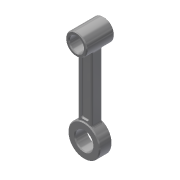
# Autodesk Inventor part: Connector Arm1
Saved by Autodesk Inventor 2022 Beta2 (Build 260130000, 130) ContinuousBuild 0
## iProperties
Shininess: 64.0
Angle Display Precision: 2
Document Length Units: 11272
Document Angle Units: 11279
Document Time Units: 11290
Document Mass Units: 11286
Document Length Units Precision: 3
Document Angle Units Precision: 2
Created: 2002-04-22
Part Number: Connector Arm1
Material: Stainless Steel, Austenitic
Document SubType Name: Modeling
Designer: Nino
Density: 8.03 g/cm^3
Appearance: Steel
Density: 0.0
Volumn: 0.0
Area: 0.0
PropertySet Name: Model Information
Control State: 0
Master: False
Checked Out: False
Author: Nino
Autodesk Inventor part; units mm, degrees
ref_plane "YZ Plane" through (0, 0, 0) normal (1, 0, 0) x (0, 1, 0)
ref_plane "XZ Plane" through (0, 0, 0) normal (0, 1, 0) x (-1, 0, 0)
sketch "Sketch1" plane through (0, 0, 0) normal (0, 0, 1) x (1, 0, 0)
  line L0 (416.0385, 369.5119) -> (416.0385, 213.9034)
  circle A0 centre (416.0385, 369.5119) radius 12.7
  circle A1 centre (416.0385, 213.9034) radius 15.875
  circle A2 centre (416.0385, 369.5119) radius 19.05
  circle A3 centre (416.0385, 213.9034) radius 28.575
  line L1 (428.7385, 355.3128) -> (428.7385, 239.5011)
  line L2 (403.3385, 355.3128) -> (403.3385, 239.5011)
  dimension "d0" = 25.4
  dimension "d1" = 31.75
  dimension "d2" = 6.35
  dimension "d3" = 12.7
  dimension "d4" = 12.7
  dimension "d5" = 12.7
  dimension "d6" = 155.6085
  constraints: 6 end point, 4 centre point, 4 point on circle, 2 coincident, 1 vertical
  measures "d0" diameter of A0
  measures "d1" diameter of A1
  measures "d2" radial gap between concentric circles of A2 A0
  measures "d3" radial gap between concentric circles of A3 A1
  measures "d4" distance between parallel lines of L2 L0
  measures "d5" distance between parallel lines of L1 L0
  measures "d6" distance of L0.start L0.end
extrude "Extrusion1" add sketch "Sketch1" along normal mid plane 19.05
ref_plane "Work Plane1" through (0, 0, 0) normal (0, 0, 1) x (1, 0, 0)
sketch "Sketch2" plane through (0, 0, 0) normal (0, 0, 1) x (1, 0, 0)
  circle A0 centre (416.0385, 369.5119) radius 12.7
  circle A1 centre (416.0385, 213.9034) radius 15.875
  circle A2 centre (416.0385, 369.5119) radius 19.05
  circle A3 centre (416.0385, 213.9034) radius 28.575
  point P0 (428.7385, 355.3128)
  point P1 (428.7385, 239.5011)
  point P2 (403.3385, 355.3128)
  point P3 (403.3385, 239.5011)
  dimension "d10" = 25.4
  dimension "d11" = 31.75
  dimension "d12" = 6.35
  dimension "d13" = 12.7
  constraints: 4 centre point, 4 point on circle
  measures "d10" diameter of A0
  measures "d11" diameter of A1
  measures "d12" radial gap between concentric circles of A2 A0
  measures "d13" radial gap between concentric circles of A3 A1
extrude "Extrusion2" add sketch "Sketch2" along normal mid plane 49.53 contours A2
extrude "Extrusion3" add sketch "Sketch2" along normal mid plane 22.352 contours A3
chamfer "Chamfer1" distance 1.524 angle 45 8 edges at (403.3385, 369.5119, 24.765) (396.9885, 369.5119, 24.765) (396.9885, 369.5119, -24.765) (403.3385, 369.5119, -24.765) (387.4635, 213.9034, 11.176) (400.1635, 213.9034, 11.176) (387.4635, 213.9034, -11.176) (400.1635, 213.9034, -11.176)
fillet "Fillet1" radius 6.35 6 edges at (428.7385, 355.3128, 0) (403.3385, 355.3128, 0) (403.3385, 239.5011, 4.7625) (403.3385, 239.5011, -4.7625) (428.7385, 239.5011, 4.7625) (428.7385, 239.5011, -4.7625)
fillet "Fillet2" radius 3.175 12 edges at (403.3385, 297.9434, 9.525) (402.9284, 354.9564, 9.525) (402.5705, 240.1482, 9.525) (403.3385, 297.9434, -9.525) (402.5705, 240.1482, -9.525) (402.9284, 354.9564, -9.525) (428.7385, 297.9434, 9.525) (429.5066, 240.1482, 9.525) (429.1487, 354.9564, 9.525) (428.7385, 297.9434, -9.525) (429.1487, 354.9564, -9.525) (429.5066, 240.1482, -9.525)
sketch "Sketch3" plane through (0, 0, 9.525) normal (0, 0, 1) x (1, 0, 0)
  arc A0 (406.5086, 353.0169) -> (425.5684, 353.0169) centre (416.0385, 369.5119) ccw projected
  line L0 (406.5135, 243.1755) -> (406.5135, 352.7114) projected
  line L1 (425.5635, 352.7114) -> (425.5635, 243.1755) projected
  line L2 (409.0535, 347.1599) -> (423.0235, 347.1599)
  line L3 (423.0235, 347.1599) -> (423.0235, 245.6534)
  line L4 (423.0235, 245.6534) -> (409.0535, 245.6534)
  line L5 (409.0535, 245.6534) -> (409.0535, 347.1599)
  circle A1 centre (416.0385, 213.9034) radius 17.399 projected
  dimension "d22" = 22.352
  dimension "d23" = 31.75
  dimension "d24" = 2.54
  dimension "d25" = 2.54
  constraints: 8 end point, 2 parallel, 1 horizontal, 1 perpendicular
  measures "d22" distance from line of A0.centre L2
  measures "d23" distance from line of A1.centre L4
  measures "d24" distance between parallel lines of L0 L5
  measures "d25" distance between parallel lines of L1 L3
extrude "Extrusion4" cut sketch "Sketch3" against normal blind 3.175 contours L2 L3 L4 L5
fillet "Fillet3" radius 3.175 4 edges at (409.0535, 245.6534, 7.9375) (423.0235, 245.6534, 7.9375) (409.0535, 347.1599, 7.9375) (423.0235, 347.1599, 7.9375)
fillet "Fillet4" radius 1.524 8 edges at (409.0535, 296.4066, 6.35) (409.9835, 246.5834, 6.35) (416.0385, 245.6534, 6.35) (422.0936, 246.5834, 6.35) (423.0235, 296.4066, 6.35) (422.0936, 346.2299, 6.35) (416.0385, 347.1599, 6.35) (409.9835, 346.2299, 6.35)
mirror "Mirror1" about plane through (0, 0, 0) normal (0, 0, 1) of "Extrusion4", "Fillet3", "Fillet4"
equation "\"d5\" = d4"
equation "\"d24\" = d25"
equation "\"d9\" = -0.5 * d7"
equation "\"d7\" = 19.05"
body "Solid1"
